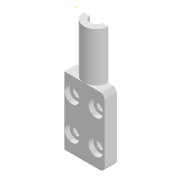
# Autodesk Inventor part: NadelHalterLose
Saved by Autodesk Inventor 2020.3 (Build 243373000, 373)
## iProperties
Created: 2021-05-31
Part Number: NadelHalterLose
Material: Generisch
Document SubType Name: Modeling
Designer: Sven
Density: 1 g/cm^3
Appearance: Vorgabe
Author: Sven
Autodesk Inventor part; units mm, degrees
ref_plane "YZ Plane" through (0, 0, 0) normal (1, 0, 0) x (0, 1, 0)
ref_plane "XZ Plane" through (0, 0, 0) normal (0, 1, 0) x (-1, 0, 0)
ref_plane "XY Plane" through (0, 0, 0) normal (0, 0, 1) x (1, 0, 0)
sketch "Skizze1" plane through (0, 0, 0) normal (0, 0, 1) x (1, 0, 0)
  circle A0 centre (3.625, -20.7) radius 1.6 projected
  circle A1 centre (3.625, -7) radius 1.6 projected
  line L0 (7.8, -27.7) -> (7.8, -25.75) projected
  line L1 (7.8, -25.75) -> (7.25, -25.75) projected
  line L2 (7.25, -25.75) -> (7.25, 0) projected
  line L3 (0, 0) -> (7.25, 0) projected
  line L4 (0, -27.7) -> (0, 0) projected
  line L5 (0, -27.7) -> (7.8, -27.7) projected
  circle A2 centre (13.375, -20.7) radius 1.6 projected
  circle A3 centre (13.375, -7) radius 1.6 projected
  line L6 (9.2, -25.75) -> (9.2, -27.7) projected
  line L7 (9.2, -27.7) -> (17, -27.7) projected
  line L8 (17, 0) -> (17, -27.7) projected
  line L9 (9.75, 0) -> (17, 0) projected
  line L10 (9.75, 0) -> (9.75, -25.75) projected
  line L11 (9.75, -25.75) -> (9.2, -25.75) projected
  line L12 (0.5, 0) -> (17, 0)
  line L13 (17, 0) -> (17, -27.7)
  line L14 (17, -27.7) -> (0.5, -27.7)
  line L15 (0.5, -27.7) -> (0.5, 0)
  dimension "d0" = 0.5
  constraints: 8 end point, 2 parallel, 1 horizontal, 1 perpendicular, 1 point on line
  measures "d0" distance between parallel lines of L4 L15
extrude "Extrusion1" add sketch "Skizze1" along normal blind 5 contours A0 | A1 | L5 L15 L3 L2 L1 L0 | L0 L1 L2 L12 L10 L11 L6 L14 | L6 L11 L10 L9 L8 L7 | A2 | A3
sketch "Skizze2" plane through (0, 0, 5) normal (0, 0, 1) x (1, 0, 0)
  circle A0 centre (3.625, -7) radius 1.6 projected
  circle A1 centre (13.375, -7) radius 1.6 projected
  circle A2 centre (13.375, -20.7) radius 1.6 projected
  circle A3 centre (3.625, -20.7) radius 1.6 projected
  point P0 (0, 0)
extrude "Extrusion2" cut sketch "Skizze2" against normal blind 10
sketch "Skizze3" plane through (0, 0, 0) normal (0, 0, -1) x (-1, 0, 0)
  line L0 (-7.25, -25.75) -> (-7.25, 0) projected
  line L1 (-9.75, 0) -> (-9.75, -25.75) projected
  line L2 (-9.75, -25.75) -> (-7.25, -25.75) projected
  line L3 (-7.25, 0) -> (-9.75, 0)
  line L4 (-17, 0) -> (-0.5, 0) projected
  point P0 (0, 0)
  dimension "d5" = 2.5
  constraints: 2 end point, 1 collinear
  measures "d5" distance of L1.end L0.start
extrude "Extrusion3" cut sketch "Skizze3" against normal blind 1.25
sketch "Skizze4" plane through (0, 0, 0) normal (0, 0, -1) x (-1, 0, 0)
  line L0 (-7.8, -27.7) -> (-7.8, -25.75) projected
  line L1 (-9.2, -25.75) -> (-9.2, -27.7) projected
  line L2 (-7.8, -27.7) -> (-9.2, -27.7)
  line L3 (-0.5, -27.7) -> (-17, -27.7) projected
  line L4 (-7.8, -25.75) -> (-9.2, -25.75)
  line L5 (-7.25, -25.75) -> (-9.75, -25.75) projected
  point P0 (0, 0)
  dimension "d8" = 1.4
  constraints: 4 end point, 2 collinear
  measures "d8" distance of L0.end L1.start
extrude "Extrusion4" cut sketch "Skizze4" against normal blind 0.7
fillet "Rundung1" radius 2 2 edges at (17, 0, 2.5) (17, -27.7, 2.5)
sketch "Skizze5" plane through (0.5, 0, 5) normal (0, 1, 0) x (1, 0, 0)
  line L0 (0, 5) -> (7.3, 5) projected
  line L1 (8.7, 5) -> (14.5, 5) projected
  arc A0 (5.5, 5) -> (10.5, 5) centre (8, 5) ccw
  line L2 (8.7, 4.3) -> (7.3, 4.3) projected
  arc A1 (3, 5) -> (13, 5) centre (8, 5) ccw
  line L3 (13, 5) -> (10.5, 5)
  line L4 (5.5, 5) -> (3, 5)
  line L5 (14.5, 0) -> (0, 0) projected
  point P0 (-0.5, 5)
  point P1 (8, 4.3)
  dimension "d12" = 2.5
  dimension "d13" = 0
  constraints: 4 end point, 4 point on circle, 4 point on line, 2 centre point, 2 collinear, 1 concentric, 1 midpoint, 1 tangent, 1 vertical alignment
  measures "d12" radius of A0
  measures "d13" distance from line of L0 A0.centre
extrude "Extrusion5" add sketch "Skizze5" along normal blind 20
sketch "Skizze7" plane through (0, 0, 5) normal (0, 0, 1) x (1, 0, 0)
  circle A0 centre (3.625, -7) radius 3
  circle A1 centre (13.375, -7) radius 3
  circle A2 centre (13.375, -20.7) radius 1.6 projected
  circle A3 centre (13.375, -20.7) radius 3
  circle A4 centre (3.625, -20.7) radius 3
  circle A5 centre (3.625, -7) radius 1.6 projected
  circle A6 centre (13.375, -7) radius 1.6 projected
  circle A7 centre (3.625, -20.7) radius 1.6 projected
  point P0 (0, 0)
  dimension "d18" = 6
  constraints: 4 centre point, 3 concentric, 3 equal radius, 1 coincident
  measures "d18" diameter of A0
extrude "Extrusion7" cut sketch "Skizze7" against normal blind 2 contours A0 | A1 | A2 | A3 | A4 | A5 | A7
sketch "Skizze8" plane through (0.5, 20, 5) normal (0, 1, 0) x (1, 0, 0)
  point P0 (-0.5, 5)
sketch "Skizze9" plane through (0.5, 20, 5) normal (0, 1, 0) x (1, 0, 0)
  line L0 (13, 5) -> (10.5, 5) projected
  arc A0 (5.5, 5) -> (10.5, 5) centre (8, 5) ccw projected
  line L1 (5.5, 5) -> (3, 5) projected
  arc A1 (3, 5) -> (13, 5) centre (8, 5) ccw projected
  circle A2 centre (8, 5) radius 5
  line L2 (5.5, 5) -> (10.5, 5)
  point P0 (-0.5, 5)
  point P1 (3, 5)
  point P2 (13, 5)
  constraints: 2 end point, 1 centre point, 1 coincident, 1 collinear
extrude "Extrusion8" add sketch "Skizze9" along normal blind 2 contours A1 L1 A0 L0 | A0 L2
equation "\"d6\" = 0.5 * d5"
equation "\"d9\" = 0.5 * d8"
